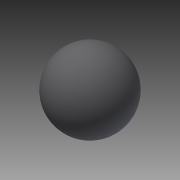
# Autodesk Inventor part: MF74ZZ Ball
Saved by Autodesk Inventor 2014 SP2 (Build 180246200, 246)
## iProperties
Created: 2019-11-12
Part Number: MF74ZZ Ball
Material: Generic
Catalog Web Link: www.cadenas.de
Description: shielded_type_zz_zzs_B-
Vendor: NSK_RB
Document SubType Name: Modeling
Designer: psadmin
Manufacturer: NSK_RB
Mass: 0.000381704 g
Surface Area: 0.0254469 cm^2
Volume: 0.000381704 cm^3
Density: 1 g/cm^3
Appearance: PSOLRGB-128-128-128
Category: PARTsolutions
Company: NSK_RB
Title: MF74ZZ Ball
Author: Cadenas PARTsolutions
PSOL_IDENT_0: {$CADENAS_DATA\23d-libs\nsk_rb\roller_bearings\deep_groove_bb\exstra_small_miniatur_bb\metric_design
PSOL_IDENT_1: _with_flange\shielded_type_zz_zzs_b_1.prj},179 {VTYP=3D},{NB=MF74ZZ Ball},{LINA=MF74ZZ Ball},{NN=shi
PSOL_IDENT_2: elded_type_zz_zzs_B},{DATE=16.01.2019 01:41:14},{GEOMDATE=04.01.2008 00:00:00},{VERSION=},{LINEID=29
PSOL_IDENT_3: 0},{WBVAR=},{WBNUMERIC=}  {NB=MF74ZZ Ball},{LINA=MF74ZZ Ball},{KT=DUMMY},{IDNR=},{STAN=},{ORDER=MF74
PSOL_IDENT_4: ZZ},{SD=4.0},{X=4.0},{D=7},{DD=7},{DD1=0.0},{D2=8.2},{DD2=8.2},{B=0.0},{B1=2.5},{CC1=0.0},{C2=0.6},{
PSOL_IDENT_5: CC2=0.6},{R=0.00},{R1=0.10},{DI1=4.80},{DI2=4.80},{SDE1=6.00},{SDE2=6.30},{CR1=255},{COR1=107},{CR2=
PSOL_IDENT_6: 26},{COR2=11.0},{LG=60000},{LO=67000},{DA=0.0},{DB=4.8},{RA=0.00},{RB=0.10},{MASS=0.35},{SC=1}
NN: shielded_type_zz_zzs_B
NB: MF74ZZ Ball
NBSYN: $ORDER. Ball
LINA: MF74ZZ Ball
ORDER: MF74ZZ
SD: 4
X: 4
D: 7
DD: 7
DD1: 0
D2: 8.2
DD2: 8.2
B: 0
B1: 2.5
CC1: 0
C2: 0.6
CC2: 0.6
R: 0
R1: 0.1
DI1: 4.8
DI2: 4.8
SDE1: 6
SDE2: 6.3
CR1: 255
COR1: 107
CR2: 26
COR2: 11
LG: 60000
LO: 67000
DA: 0
DB: 4.8
RA: 0
RB: 0.1
MASS: 0.35
SC: 1
SUPPLIER: NSK_RB
ARTICLENO: MF74ZZ Ball
BOMINFO: MF74ZZ Ball
CREATOR: CADENAS GmbH
Autodesk Inventor part; units mm, degrees
sketch "Sketch_1" plane through (0, 0, 0) normal (0, 0, 1) x (1, 0, 0)
  line L0 (0.45, 0) -> (-0.45, 0)
  arc A0 (0.45, 0) -> (-0.45, 0) centre (0, 0) ccw
  line L1 (0.45, 0) -> (-0.45, 0)
  constraints: 4 end point, 2 point on circle, 1 centre point
revolve "Revolution1" add sketch "Sketch_1" angle 360 about axis through (0.45, 0, 0) along (1, 0, 0)
ref_plane "ip_st_1_XY" through (0, 0, 0) normal (-1, 0, 0) x (0, 0, -1)
ref_plane "ip_st_1_YZ" through (0, 0, 0) normal (0, 0, -1) x (0, -1, 0)
ref_plane "ip_st_1_ZX" through (0, 0, 0) normal (0, -1, 0) x (-1, 0, 0)
body "Solid1"
